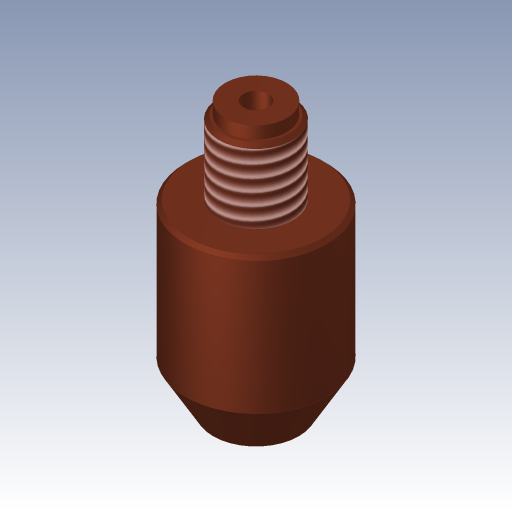
# Autodesk Inventor part: BT002_huenin20_23
Saved by Autodesk Inventor 2023.3 (Build 273359000, 359)
## iProperties
Company: HTBLA Kaindorf
RuleStatus: InUse
Created: 2023-08-12
Part Number: BT002_huenin20_23
Project: Fiberprinter-Hotend
Material: Kupfer
Description: Nozzel_extender
Document SubType Name: Modeling
Designer: huenin20
Density: 8.94 g/cm^3
Appearance: Kupfer - satiniert
Mass: 13.0418 g
Surface Area: 9.70927 cm^2
Volume: 1.45881 cm^3
AfterDocNew0: iProperties-Editor_aufrufen
Author: nicob
Keywords: 2023
Autodesk Inventor part; units mm, degrees
ref_plane "YZ Plane" through (0, 0, 0) normal (1, 0, 0) x (0, 1, 0)
ref_plane "XZ Plane" through (0, 0, 0) normal (0, 1, 0) x (-1, 0, 0)
ref_plane "XY Plane" through (0, 0, 0) normal (0, 0, 1) x (1, 0, 0)
sketch "Skizze3" plane through (0, 0, 0) normal (1, 0, 0) x (0, 1, 0)
  line L0 (0, 0) -> (0, 30.5982)
  line L1 (0, 0) -> (-3.5, 0)
  line L2 (-3.5, 0) -> (-5.75, 3.8971)
  line L3 (-5.75, 3.8971) -> (-5.75, 15)
  line L4 (-5.75, 15) -> (-3, 15)
  line L5 (-3, 15) -> (-3, 21)
  line L6 (-3, 21) -> (-2.5, 21)
  line L7 (-2.5, 21) -> (-2.5, 22)
  line L8 (-2.5, 22) -> (0, 22)
  line L9 (-1, 22) -> (-1, 0)
  point P0 (-2.75, 21)
  dimension "d7" = 7
  dimension "d8" = 15
  dimension "d9" = 11.5
  dimension "d10" = 6
  dimension "d11" = 6
  dimension "d12" = 5
  dimension "d13" = 1
  dimension "d14" = 120
  dimension "d15" = 2
  constraints: 20 end point, 6 perpendicular, 3 point on line, 2 horizontal, 1 midpoint, 1 vertical
  measures "d7" diameter of L1.end L0
  measures "d8" vertical distance of L1.end L3.end
  measures "d9" diameter of L3 L0
  measures "d10" distance of L4.end L5.end
  measures "d11" diameter of L5 L0
  measures "d12" diameter of L7 L0
  measures "d13" distance from line of point (-2.75, 21) L8
  measures "d14" angle of L1 L2
  measures "d15" diameter of L9 L0
revolve "Umdrehung1" add sketch "Skizze3" angle 360 about axis through (0, 0, 0) along (0, 0, 1) contours L1 L2 L3 L4 L5 L6 L7 L8 L9
thread "Gewinde1" size "M6x1" class "6g" standard "ISO Metric profile" length 15
chamfer "Fase1" distance 0.3 angle 45 2 edges at (0, 3, 21) (0, 5.75, 15)
sketch "Skizze4" plane through (0, 0, 0) normal (0, 0, -1) x (-1, 0, 0)
  circle A0 centre (0, 0) radius 1 projected
hole "Bohrung1" at (0, 0, 0) direction (0, 0, 1) diameter 4.917 depth 5 thread size "M6x1" class "6H" standard "ISO Metric profile"
equation "\"d8\" = Länge"
equation "\"Länge\" = 15"
